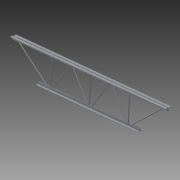
# Autodesk Inventor part: Truss
Saved by Autodesk Inventor 2013 (Build 170138000, 138)
## iProperties
Created: 2010-06-17
Part Number: Truss
Document SubType Name: Modeling
Designer: taylorm
Density: 1 g/cm^3
Material: Generic
Author: taylorm
Autodesk Inventor part; units mm, degrees
sketch "Sketch5" plane through (0, 0, 0) normal (1, 0, 0) x (0, 1, 0)
  line L0 (661.7091, 87.6367) -> (661.7091, 11.6367)
  line L1 (661.7091, 11.6367) -> (585.7091, 11.6367)
  line L2 (585.7091, 11.6367) -> (585.7091, 18.0367)
  line L3 (585.7091, 18.0367) -> (655.3091, 18.0367)
  line L4 (655.3091, 18.0367) -> (655.3091, 87.6367)
  line L5 (655.3091, 87.6367) -> (661.7091, 87.6367)
  line L6 (661.7091, 87.6367) -> (661.7091, 11.6367)
  line L7 (661.7091, -89.9633) -> (661.7091, -13.9633)
  line L8 (661.7091, -13.9633) -> (585.7091, -13.9633)
  line L9 (585.7091, -13.9633) -> (585.7091, -20.3633)
  line L10 (585.7091, -20.3633) -> (655.3091, -20.3633)
  line L11 (655.3091, -20.3633) -> (655.3091, -89.9633)
  line L12 (655.3091, -89.9633) -> (661.7091, -89.9633)
  line L13 (-214.2909, 11.95) -> (-214.2909, 5.55)
  line L14 (-214.2909, 5.55) -> (-278.2909, 5.55)
  line L15 (-278.2909, 5.55) -> (-278.2909, 69.55)
  line L16 (-278.2909, 69.55) -> (-271.8909, 69.55)
  line L17 (-271.8909, 69.55) -> (-271.8909, 11.95)
  line L18 (-271.8909, 11.95) -> (-214.2909, 11.95)
  line L19 (-214.2909, -9.6424) -> (-278.2909, -9.6424)
  line L20 (-278.2909, -9.6424) -> (-278.2909, -73.6424)
  line L21 (-278.2909, -73.6424) -> (-271.8909, -73.6424)
  line L22 (-271.8909, -73.6424) -> (-271.8909, -16.0424)
  line L23 (-271.8909, -16.0424) -> (-214.2909, -16.0424)
  line L24 (-214.2909, -16.0424) -> (-214.2909, -9.6424)
  point P0 (0, 0)
  dimension "d6" = 6.4
  dimension "d7" = 6.4
  dimension "d8" = 76
  dimension "d9" = 76
  dimension "d11" = 6.4
  dimension "d12" = 6.4
  dimension "d13" = 64
  dimension "d14" = 64
  dimension "d15" = 64
  dimension "d16" = 6.4
  dimension "d17" = 800
  constraints: 50 end point, 12 parallel, 5 perpendicular, 3 collinear, 1 vertical
  measures "d6" distance between parallel lines of L0 L4
  measures "d7" distance between parallel lines of L1 L3
  measures "d8" distance between parallel lines of L1 L5
  measures "d9" distance between parallel lines of L2 L0
  measures "d11" distance between parallel lines of L14 L18
  measures "d12" distance between parallel lines of L17 L15
  measures "d13" distance between parallel lines of L14 L16
  measures "d14" distance from line of L15 L13.start
  measures "d15" distance from line of L20.end L19
  measures "d16" distance between parallel lines of L19 L23
  measures "d17" distance from line of L13.start L2
extrude "Extrusion1" add sketch "Sketch5" against normal blind 4600 contours L0 L1 L2 L3 L4 L5 | L12 L11 L10 L9 L8 L7
sketch "Sketch11" plane through (0, 0, 0) normal (0, 0, 1) x (1, 0, 0)
  line L0 (0, 655.3091) -> (0, 585.7091) projected
  line L1 (-4600, 655.3091) -> (-4600, 585.7091) projected
  point P0 (0, 0)
  point P1 (-800, 451.916)
  point P2 (-100, 451.916)
  point P3 (-2300, 451.916)
  point P4 (-1150, 451.916)
  point P5 (-3450, 451.916)
  point P6 (-4500, 451.916)
  dimension "d38" = 800
  dimension "d46" = 100
  dimension "d47" = 1150
  dimension "d48" = 2300
  dimension "d49" = 1150
  dimension "d50" = 1150
  dimension "d51" = 100
  measures "d38" distance from line of L0 point (-800, 451.916)
  measures "d46" distance from line of L0 point (-100, 451.916)
  measures "d47" distance from line of L0 point (-1150, 451.916)
  measures "d48" distance from line of L0 point (-2300, 451.916)
  measures "d49" distance from line of L1 point (-3450, 451.916)
  measures "d50" distance of point (-2300, 451.916) point (-3450, 451.916)
  measures "d51" distance from line of L1 point (-4500, 451.916)
ref_plane "Work Plane3" through (-800, 451.916, 0) normal (1, 0, 0) x (0, 1, 0)
sketch "Sketch12" plane through (-800, 451.916, 0) normal (1, 0, 0) x (0, 1, 0)
  line L0 (203.3931, 18.0367) -> (133.7931, 18.0367) projected
  line L1 (203.3931, 87.6367) -> (203.3931, 18.0367) projected
  line L2 (209.7931, 11.6367) -> (209.7931, 87.6367) projected
  line L3 (209.7931, -13.9633) -> (133.7931, -13.9633) projected
  line L4 (133.7931, -20.3633) -> (203.3931, -20.3633) projected
  line L5 (209.7931, -89.9633) -> (209.7931, -13.9633) projected
  line L6 (-526.2069, 11.6367) -> (-590.2069, 11.6367)
  line L7 (-590.2069, 11.6367) -> (-590.2069, 75.6367)
  line L8 (-590.2069, 75.6367) -> (-583.8069, 75.6367)
  line L9 (-583.8069, 75.6367) -> (-583.8069, 18.0367)
  line L10 (-583.8069, 18.0367) -> (-526.2069, 18.0367)
  line L11 (-526.2069, 18.0367) -> (-526.2069, 11.6367)
  line L12 (133.7931, 11.6367) -> (209.7931, 11.6367) projected
  line L13 (-526.2069, -13.9633) -> (-590.2069, -13.9633)
  line L14 (-590.2069, -13.9633) -> (-590.2069, -77.9633)
  line L15 (-590.2069, -77.9633) -> (-583.8069, -77.9633)
  line L16 (-583.8069, -77.9633) -> (-583.8069, -20.3633)
  line L17 (-583.8069, -20.3633) -> (-526.2069, -20.3633)
  line L18 (-526.2069, -20.3633) -> (-526.2069, -13.9633)
  point P0 (-451.916, 0)
  dimension "d39" = 64
  dimension "d40" = 64
  dimension "d41" = 6.4
  dimension "d42" = 800
  dimension "d43" = 64
  constraints: 24 end point, 7 collinear, 7 parallel, 5 perpendicular
  measures "d39" distance of L6.end L7.end
  measures "d40" distance of L6.end L6.start
  measures "d41" distance between parallel lines of L7 L9
  measures "d42" distance between parallel lines of L7 L2
  measures "d43" distance of L13.end L14.end
extrude "Extrusion3" add sketch "Sketch12" against normal blind 3000
ref_plane "Work Plane4" through (-2300, 451.916, 0) normal (1, 0, 0) x (0, 1, 0)
sketch "Sketch13" plane through (-2300, 451.916, 0) normal (1, 0, 0) x (0, 1, 0)
  line L0 (133.7931, 11.6367) -> (209.7931, 11.6367) projected
  line L1 (209.7931, -13.9633) -> (133.7931, -13.9633) projected
  line L2 (-526.2069, -13.9633) -> (-590.2069, -13.9633) projected
  line L3 (-526.2069, 11.6367) -> (-590.2069, 11.6367) projected
  line L4 (203.3931, 0) -> (133.7931, 0) projected
  line L5 (209.7931, -13.9633) -> (-590.2069, -13.9633)
  line L6 (-590.2069, -13.9633) -> (-590.2069, -1.1633)
  line L7 (-590.2069, -1.1633) -> (209.7931, -1.1633)
  line L8 (209.7931, -1.1633) -> (209.7931, -13.9633)
  point P0 (-451.916, 0)
  dimension "d52" = 12.8
  dimension "d53" = 800
  constraints: 8 end point, 2 parallel, 2 perpendicular
  measures "d52" distance between parallel lines of L5 L7
  measures "d53" distance from line of L6.end L8
revolve "Revolution3" add sketch "Sketch13" angle 360 about axis through (-2300, -138.2909, -1.1633) along (0, 1, 0)
ref_plane "Work Plane5" through (-1150, 451.916, 0) normal (1, 0, 0) x (0, 1, 0)
sketch "Sketch14" plane through (-1150, 451.916, 0) normal (1, 0, 0) x (0, 1, 0)
  line L0 (209.7931, -13.9633) -> (133.7931, -13.9633) projected
  line L1 (203.3931, 0) -> (133.7931, 0) projected
  line L2 (209.7931, -13.9633) -> (-590.2069, -13.9633) projected
  line L3 (209.7931, 11.6367) -> (209.7931, -13.9633) projected
  line L4 (-590.2069, 11.6367) -> (-590.2069, -13.9633) projected
  line L5 (209.7931, -13.9633) -> (-590.2069, -13.9633)
  line L6 (-590.2069, -13.9633) -> (-590.2069, -1.1633)
  line L7 (-590.2069, -1.1633) -> (209.7931, -1.1633)
  line L8 (209.7931, -13.9633) -> (209.7931, -1.1633)
  point P0 (-451.916, 0)
  dimension "d55" = 12.8
  constraints: 8 end point, 2 midpoint, 1 collinear, 1 perpendicular
  measures "d55" distance between parallel lines of L5 L7
revolve "Revolution4" add sketch "Sketch14" angle 360 about axis through (-1150, -138.2909, -1.1633) along (0, 1, 0)
ref_plane "Work Plane6" through (-3450, 451.916, 0) normal (1, 0, 0) x (0, 1, 0)
sketch "Sketch15" plane through (-3450, 451.916, 0) normal (1, 0, 0) x (0, 1, 0)
  line L0 (209.7931, -13.9633) -> (-590.2069, -13.9633) projected
  line L1 (209.7931, 11.6367) -> (-590.2069, 11.6367) projected
  line L2 (209.7931, 11.6367) -> (209.7931, -13.9633) projected
  line L3 (209.7931, 11.6367) -> (-590.2069, 11.6367)
  line L4 (-590.2069, 11.6367) -> (-590.2069, -1.1633)
  line L5 (-590.2069, -1.1633) -> (209.7931, -1.1633)
  line L6 (209.7931, 11.6367) -> (209.7931, -1.1633)
  point P0 (-451.916, 0)
  dimension "d57" = 12.8
  dimension "d58" = 800
  constraints: 8 end point, 2 perpendicular, 1 collinear, 1 midpoint
  measures "d57" distance between parallel lines of L3 L5
  measures "d58" distance between parallel lines of L2 L4
revolve "Revolution5" add sketch "Sketch15" angle 360 about axis through (-3450, -138.2909, -1.1633) along (0, 1, 0)
sketch "Sketch16" plane through (0, 0, 0) normal (1, 0, 0) x (0, 1, 0)
  line L0 (661.1435, -1.1633) -> (582.6816, -1.1633)
  line L1 (585.7091, 11.6367) -> (661.7091, 11.6367) projected
  line L2 (-138.2909, -13.9633) -> (-138.2909, 11.6367) projected
  line L3 (-74.2909, -13.9633) -> (-138.2909, -13.9633) projected
  line L4 (-138.2909, 11.6367) -> (-138.2909, -13.9633) projected
  line L5 (-74.2909, 11.6367) -> (-138.2909, 11.6367) projected
  line L6 (661.7091, -13.9633) -> (661.7091, 11.6367) projected
  line L7 (661.7091, 11.6367) -> (585.7091, 11.6367) projected
  line L8 (661.7091, 11.6367) -> (661.7091, -13.9633) projected
  line L9 (661.7091, -13.9633) -> (585.7091, -13.9633) projected
  point P0 (0, 0)
  dimension "d60" = 12.8
  constraints: 2 end point, 1 horizontal
  measures "d60" distance between parallel lines of L1 L0
ref_plane "Work Plane7" through (0, 661.1435, -1.1633) normal (0, 0, 1) x (1, 0, 0)
sketch "Sketch17" plane through (0, 661.1435, -1.1633) normal (0, 0, 1) x (1, 0, 0)
  line L0 (-4600, -5.8344) -> (-4600, -75.4344) projected
  line L1 (0, -75.4344) -> (-4600, -75.4344) projected
  line L2 (-3462.8, -799.4344) -> (-3462.8, 0.5656) projected
  line L3 (-4500, -5.8344) -> (-3462.8, -799.4344)
  line L4 (-4500, -5.8344) -> (-4507.7781, -16)
  line L5 (-4507.7781, -16) -> (-3488.1909, -796.1239)
  line L6 (-3488.1909, -796.1239) -> (-3480.4128, -785.9582)
  point P0 (0, -661.1435)
  dimension "d61" = 100
  dimension "d62" = 12.8
  constraints: 8 end point, 2 perpendicular, 1 parallel, 1 point on line
  measures "d61" distance from line of L3.start L0
  measures "d62" distance between parallel lines of L3 L5
revolve "Revolution6" add sketch "Sketch17" angle 360 about axis through (-4507.7781, 645.1435, -1.1633) along (0.7941926, -0.6076661, 0) contours L3 L6 L5 L1 | L1 L5 L4 L3
sketch "Sketch18" plane through (0, 661.1435, -1.1633) normal (0, 0, 1) x (1, 0, 0)
  line L0 (-3437.2, -799.4344) -> (-3437.2, 0.5656) projected
  line L1 (-2312.8, 0.5656) -> (-2312.8, -799.4344) projected
  line L2 (-2300, 0.5656) -> (-3450, 0.5656) projected
  line L3 (-3437.2, -799.4344) -> (-3450, -799.4344) projected
  line L4 (-3437.2, -799.4344) -> (-2862.2, 0.5656)
  line L5 (-2862.2, 0.5656) -> (-2851.8062, -6.9049)
  line L6 (-2851.8062, -6.9049) -> (-3426.8062, -806.9049)
  line L7 (-3426.8062, -806.9049) -> (-3437.2, -799.4344)
  line L8 (-2851.8062, -6.9049) -> (-2300, -799.4344)
  line L9 (-2300, -799.4344) -> (-2289.4954, -792.1205)
  line L10 (-2289.4954, -792.1205) -> (-2827.8229, -18.9497)
  line L11 (-2827.8229, -18.9497) -> (-2838.3275, -26.2636)
  line L12 (-2827.8229, -18.9497) -> (-2821.0836, -28.629)
  point P0 (0, -661.1435)
  dimension "d64" = 575
  dimension "d65" = 12.8
  dimension "d66" = 12.8
  constraints: 18 end point, 4 perpendicular, 3 point on line, 2 parallel
  measures "d64" distance from line of L4.end L0
  measures "d65" distance between parallel lines of L6 L4
  measures "d66" distance between parallel lines of L10 L8
revolve "Revolution7" add sketch "Sketch18" angle 360 about axis through (-2851.8062, 654.2386, -1.1633) along (-0.583636, -0.8120154, 0) contours L4 L5 L6 L7
sketch "Sketch19" plane through (0, 661.1435, -1.1633) normal (0, 0, 1) x (1, 0, 0)
  line L0 (-2851.8062, -6.9049) -> (-2862.2, 0.5656) projected
  line L1 (-2312.8, -799.4344) -> (-2300, -799.4344) projected
  line L2 (-2306.4, -799.4344) -> (-2862.2, 0.5656)
  line L3 (-2862.2, 0.5656) -> (-2872.712, -6.7376)
  line L4 (-2862.2, 0.5656) -> (-2872.712, -6.7376)
  line L5 (-2872.712, -6.7376) -> (-2316.912, -806.7376)
  line L6 (-2316.912, -806.7376) -> (-2306.4, -799.4344)
  point P0 (0, -661.1435)
  dimension "d68" = 12.8
  constraints: 10 end point, 2 equal length, 2 perpendicular, 1 midpoint
  measures "d68" distance between parallel lines of L2 L5
revolve "Revolution8" add sketch "Sketch19" angle 360 about axis through (-2872.712, 654.4059, -1.1633) along (0.5705651, -0.8212524, 0)
sketch "Sketch20" plane through (0, 661.1435, -1.1633) normal (0, 0, 1) x (1, 0, 0)
  line L0 (-2287.2, 0.5656) -> (-2287.2, -799.4344) projected
  line L1 (-2287.2, -799.4344) -> (-1712.2, 0.5656)
  line L2 (-1712.2, 0.5656) -> (-1701.8062, -6.9049)
  line L3 (-1701.8062, -6.9049) -> (-2259.6243, -782.9997)
  line L4 (-2259.6243, -782.9997) -> (-2270.0181, -775.5292)
  point P0 (0, -661.1435)
  dimension "d70" = 575
  dimension "d71" = 12.8
  constraints: 8 end point, 2 parallel, 1 perpendicular, 1 point on line
  measures "d70" distance from line of L1.end L0
  measures "d71" distance between parallel lines of L3 L1
revolve "Revolution9" add sketch "Sketch20" angle 360 about axis through (-1701.8062, 654.2386, -1.1633) along (-0.583636, -0.8120154, 0)
sketch "Sketch21" plane through (0, 661.1435, -1.1633) normal (0, 0, 1) x (1, 0, 0)
  line L0 (-1701.8062, -6.9049) -> (-1150, -799.4344)
  line L1 (-1150, -799.4344) -> (-1139.4954, -792.1205)
  line L2 (-1139.4954, -792.1205) -> (-1679.8588, -16.0257)
  line L3 (-1679.8588, -16.0257) -> (-1690.3634, -23.3396)
  point P0 (0, -661.1435)
  point P1 (-2259.6243, -782.9997)
  dimension "d73" = 12.8
  constraints: 8 end point, 2 perpendicular, 1 parallel, 1 point on line
  measures "d73" distance between parallel lines of L2 L0
revolve "Revolution10" add sketch "Sketch21" angle 360 about axis through (-1701.8062, 654.2386, -1.1633) along (0.5714003, -0.8206715, 0)
sketch "Sketch22" plane through (0, 661.1435, -1.1633) normal (0, 0, 1) x (1, 0, 0)
  line L0 (0, 0.5656) -> (0, -75.4344) projected
  line L1 (0, -5.8344) -> (0, -75.4344) projected
  line L2 (-1150, -799.4344) -> (-1137.2, -799.4344) projected
  line L3 (-1137.2, -799.4344) -> (-100, 0.5656)
  line L4 (-100, 0.5656) -> (-92.1825, -9.5698)
  line L5 (-92.1825, -9.5698) -> (-1102.8811, -789.1291)
  line L6 (-1102.8811, -789.1291) -> (-1110.6986, -778.9936)
  point P0 (0, -661.1435)
  dimension "d75" = 100
  dimension "d76" = 12.8
  constraints: 8 end point, 2 parallel, 1 perpendicular, 1 point on line
  measures "d75" distance from line of L1 L3.end
  measures "d76" distance between parallel lines of L5 L3
revolve "Revolution11" add sketch "Sketch22" angle 360 about axis through (-92.1825, 651.5737, -1.1633) along (-0.7918287, -0.6107433, 0)
body "Solid2"
